# Autodesk Inventor part: V-Belt
Saved by Autodesk Inventor 2014 (Build 180170000, 170)
## iProperties
Created: 2017-06-15
Part Number: V-Belt
Material: Rubber
Document SubType Name: Modeling
Designer: RMcComber
Density: 0.93 g/cm^3
Appearance: Rubber - Black - Version 1.1
CustomPartVersion: 1
Author: RMcComber
Autodesk Inventor part; units mm, degrees
ref_plane "YZ Plane" through (0, 0, 0) normal (1, 0, 0) x (0, 1, 0)
ref_plane "XZ Plane" through (0, 0, 0) normal (0, 1, 0) x (-1, 0, 0)
sketch "Sketch Path" plane through (0, 0, 0) normal (0, 0, 1) x (1, 0, 0)
  arc A0 (45, 40.64) -> (45, -40.64) centre (45, 0) ccw
  arc A1 (264.0357, -40.64) -> (264.0357, 40.64) centre (264.0357, 0) ccw
  line L0 (264.0357, -40.64) -> (45, -40.64)
  line L1 (45, 40.64) -> (264.0357, 40.64)
  constraints: 4 end point, 4 point on circle, 2 centre point
ref_plane "Cross Section Plane" through (45, -40.64, 0) normal (1, 0, 0) x (0, 0, 1)
sketch "Cross Section" plane through (45, -40.64, 0) normal (1, 0, 0) x (0, 0, 1)
  line L0 (0, 2.6822) -> (0, -5.2553) construction
  line L1 (-5.3086, 0) -> (5.3086, 0) construction
  line L2 (-6.2848, 2.6822) -> (6.2848, 2.6822)
  line L3 (6.2848, 2.6822) -> (3.3958, -5.2553)
  line L4 (3.3958, -5.2553) -> (-3.3958, -5.2553)
  line L5 (-3.3958, -5.2553) -> (-6.2848, 2.6822)
  point P0 (0, 0)
  point P1 (0, 0)
  point P2 (0, 0)
  dimension "d0" = 10.6172
  dimension "d1" = 2.6822
  dimension "d2" = 40
  dimension "d3" = 7.9375
  constraints: 12 end point, 3 midpoint, 2 parallel, 2 point on line, 1 coincident, 1 perpendicular, 1 vertical, 1 other
  measures "d0" distance of L1.start L1.end
  measures "d1" distance between parallel lines of L2 L1
  measures "d2" angle of L5 L3
  measures "d3" distance between parallel lines of L4 L2
sweep "Belt" add profiles "Cross Section" path "Sketch Path"
equation "\"d0\" = da_Bw"
equation "\"d1\" = da_Hw"
equation "\"d2\" = da_Alfa"
equation "\"d3\" = da_H"
equation "\"da_Alfa\" = 40deg"
equation "\"da_H\" = 7.9375"
equation "\"da_Bw\" = 10.6172"
equation "\"da_Hw\" = 2.6822"
body "Solid1"
